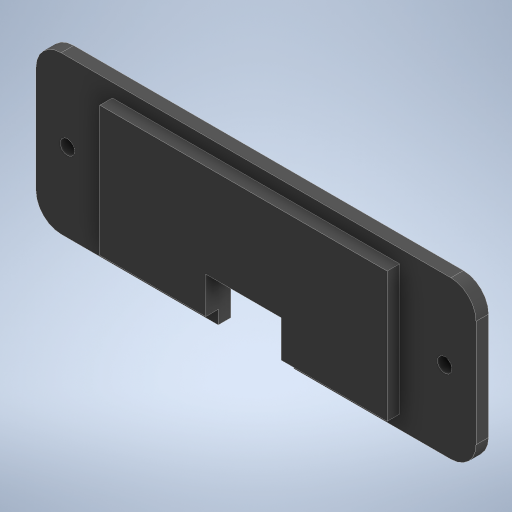
# Autodesk Inventor part: UltrasonicSensorMountTest_backplate
Saved by Autodesk Inventor 2024.2 (Build 282272000, 272)
## iProperties
Created: 2024-04-02
Part Number: UltrasonicSensorMountTest_backplate
Material: Generic
Document SubType Name: Modeling
Designer: ringl
Density: 1 g/cm^3
Appearance: Default(1)
Author: ringl
Autodesk Inventor part; units mm, degrees
ref_plane "YZ Plane" through (0, 0, 0) normal (1, 0, 0) x (0, 1, 0)
ref_plane "XZ Plane" through (0, 0, 0) normal (0, 1, 0) x (-1, 0, 0)
sketch "Sketch1" plane through (0, 0, 0) normal (0, 0, 1) x (1, 0, 0)
  line L0 (0, 0) -> (50, 0)
  line L1 (50, 0) -> (50, -25)
  line L2 (50, -25) -> (0, -25)
  line L3 (0, -25) -> (0, 0)
  line L4 (50, 0) -> (60, 0)
  line L5 (60, -25) -> (50, -25)
  line L6 (0, -25) -> (-10, -25)
  line L7 (-10, 0) -> (0, 0)
  circle A0 centre (55, -12.5) radius 1.15
  circle A1 centre (-5, -12.5) radius 1.15
  line L8 (-10, 0) -> (-10, -25)
  line L9 (60, 0) -> (60, -25)
  point P0 (60, -12.5)
  point P1 (-10, -12.5)
  dimension "d0" = 50
  dimension "d1" = 25
  dimension "d19" = 10
  dimension "d20" = 10
  dimension "d21" = 2.3
  dimension "d22" = 2.3
  dimension "d37" = 12.5
  dimension "d38" = 12.5
  dimension "d39" = 12.5
  dimension "d40" = 5
  dimension "d41" = 5
  dimension "d42" = 12.5
  dimension "d43" = 12.5
  constraints: 20 end point, 2 centre point, 2 midpoint, 2 parallel, 2 vertical, 1 coincident, 1 horizontal, 1 horizontal alignment, 1 perpendicular
  measures "d0" distance of L1.end L2.end
  measures "d1" distance of L0.end L1.end
  measures "d19" distance of L5.start L1.end
  measures "d20" distance from line of L7.start L3
  measures "d21" diameter of A0
  measures "d22" diameter of A1
  measures "d37" vertical distance of point (0, 0) A1.centre
  measures "d38" vertical distance of L4.end A0.centre
  measures "d39" vertical distance of L5.start A0.centre
  measures "d40" distance of point (60, -12.5) A0.centre
  measures "d41" distance of A1.centre point (-10, -12.5)
  measures "d42" vertical distance of L7.start A1.centre
  measures "d43" vertical distance of L6.end A1.centre
extrude "Extrusion1" add sketch "Sketch1" along normal blind 2
sketch "Sketch4" plane through (0, 0, 2) normal (0, 0, 1) x (1, 0, 0)
  line L0 (2.15, -22.85) -> (47.85, -22.85)
  line L1 (47.85, -22.85) -> (47.85, -2.15)
  line L2 (47.85, -2.15) -> (2.15, -2.15)
  line L3 (2.15, -2.15) -> (2.15, -22.85)
  line L4 (60, -25) -> (60, 0) projected
  point P0 (0, 0)
  point P1 (2.15, -12.5)
  point P2 (50, -25)
  dimension "d25" = 20.7
  dimension "d26" = 2.15
  dimension "d27" = 45.7
  dimension "d44" = 12.15
  constraints: 8 end point, 2 parallel, 1 horizontal, 1 midpoint, 1 perpendicular
  measures "d25" distance between parallel lines of L2 L0
  measures "d26" distance from line of point (0, 0) L2
  measures "d27" distance from line of L1 point (2.15, -12.5)
  measures "d44" distance between parallel lines of L1 L4
ref_plane "Work Plane1" through (0, 0, 4) normal (0, 0, 1) x (1, 0, 0)
sketch "Sketch5" plane through (0, 0, 4) normal (0, 0, 1) x (1, 0, 0)
  line L0 (31, -25) -> (19, -25)
  line L1 (19, -25) -> (19, -17)
  line L2 (19, -17) -> (31, -17)
  line L3 (31, -17) -> (31, -25)
  line L4 (-10, -25) -> (60, -25) projected
  line L5 (-10, 0) -> (-10, -25) projected
  point P0 (0, 0)
  dimension "d32" = 12
  dimension "d33" = 8
  dimension "d50" = 29
  constraints: 8 end point, 2 parallel, 1 horizontal, 1 perpendicular, 1 point on line
  measures "d32" distance of L1.end L2.end
  measures "d33" distance of L2.end L0.start
  measures "d50" distance between parallel lines of L5 L1
fillet "Fillet1" radius 4 4 edges at (-10, 0, 1) (60, 0, 1) (-10, -25, 1) (60, -25, 1)
extrude "Extrusion6" add sketch "Sketch4" along normal blind 2
extrude "Extrusion7" cut sketch "Sketch5" against normal through all
body "Solid1"
